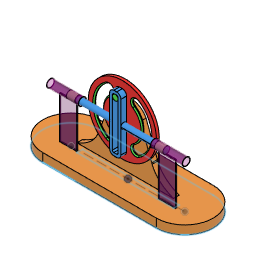
SCOTCH YOKE MECHANISM (Autodesk Fusion 360 design; units mm, degrees)
Autodesk Fusion 360 part; units mm, degrees
note: some values were not read from the file. Chosen so that the rebuilt part matches the saved one: that a step has no effect; which face or edge a step refers to; which pieces of a blend or face edit are solid. Set by a fixed rule: which sketch regions a step uses.
sketch "Holder stand" plane through (0, 0, 0) normal (0, 1, 0) x (1, 0, 0) in component "Holder stand"
  line L0 (-100, -50) -> (100, -50)
  arc A0 (100, -50) -> (100, 50) centre (100, 0) ccw
  line L1 (100, 50) -> (-100, 50)
  arc A1 (-100, 50) -> (-100, -50) centre (-100, 0) ccw
  line L2 (-100, 0) -> (100, 0) construction
  constraint tangent L0 A0
  constraint tangent A0 L1
  constraint parallel L0 L1
  constraint tangent L1 A1
  constraint tangent L0 A1
  constraint horizontal L2
  constraint midpoint L2 origin
extrude "Extrude1" add sketch "Holder stand" along normal blind 15 makes body 1 in component "Holder stand"
sketch "Crank holder hole" plane through (0, 0, 0) normal (0, 1, 0) x (1, 0, 0) in component "Holder stand"
  line L0 (-85, -5) -> (85, -5)
  line L1 (85, -5) -> (85, 5)
  line L2 (85, 5) -> (-85, 5)
  line L3 (-85, 5) -> (-85, -5)
  constraint horizontal L0
  constraint vertical L1
  constraint horizontal L2
  constraint vertical L3
extrude "Extrude2" cut sketch "Crank holder hole" along normal blind 15 bodies 1 in component "Holder stand"
sketch "Holder" plane through (0, 0, 0) normal (0, 0, 1) x (1, 0, 0) in component " Crank Holder"
  line L0 (0, 15) -> (0, 100.6882)
  line L1 (-26.793, 103.552) -> (-47.4731, 48.405)
  line L2 (-60, 15) -> (0, 15)
  line L3 (-60, 15) -> (-85, 15)
  spline S0 degree 5 poles (-85, 15) (-82.4129, 16.0125) (-77.423, 18.1587) (-70.4912, 21.7416) (-62.3731, 27.258) (-55.1239, 34.5502) (-50.7724, 41.0341) (-48.3509, 46.0734) (-47.1533, 49.2041) (-46.8071, 50.181) knots 0 0 0 0 0 0 0.1 0.2 0.3 0.4 0.444391 0.444391 0.444391 0.444391 0.444391 0.444391
  line L4 (-48.7805, 44.6118) -> (-44.8337, 55.7502)
  line L5 (26.793, 103.552) -> (47.4731, 48.405)
  spline S1 degree 5 poles (85, 15) (82.4129, 16.0125) (77.423, 18.1587) (70.4912, 21.7416) (62.3731, 27.258) (55.1239, 34.5502) (50.7724, 41.0341) (48.3509, 46.0734) (47.1533, 49.2041) (46.8071, 50.181) knots 0 0 0 0 0 0 0.1 0.2 0.3 0.4 0.444391 0.444391 0.444391 0.444391 0.444391 0.444391
  line L6 (-91.3253, 12.5245) -> (-78.6747, 17.4755)
  line L7 (91.3253, 12.5245) -> (78.6747, 17.4755)
  line L8 (48.7805, 44.6118) -> (44.8337, 55.7502)
  line L9 (60, 15) -> (0, 15)
  line L10 (60, 15) -> (85, 15)
  arc A0 (29.0974, 97.4069) -> (-29.0974, 97.4069) centre (0, 90) ccw
  point P0 (-46.8073, 50.1805)
  point P1 (46.8073, 50.1805)
  constraint vertical L0
  constraint perpendicular L0 L2
  constraint coincident L1 P0
  constraint parallel L2 L3
  constraint coincident L1 S0.end
  constraint midpoint S0.end L4
  constraint coincident S0 L1.end
  constraint midpoint L3.end L6
  constraint symmetric L2.end L0 L9.end
  constraint symmetric L0 L2.start L9.start
  constraint symmetric L0 L3.end S1.start
  constraint symmetric L0 P0 P1
  constraint symmetric L0 S0.end S1.end
  constraint symmetric L0 L4.start L8.start
  constraint symmetric L0 L4.end L8.end
  constraint symmetric L0 L1.end L5.end
  constraint symmetric L0 L6.start L7.start
  constraint symmetric L0 L6.end L7.end
  constraint coincident L0 A0.centre
  constraint coincident L1.start A0
  constraint coincident L5.start A0
  constraint coincident L5 A0.start
  constraint coincident L1 A0.end
extrude "Extrude1'" add sketch "Holder" along normal mid plane 10 separate body contours L1 L2 L3 S0 L5 S1 L9 L10 A0 makes body 2 in component " Crank Holder"
extrude "Extrude2'" add 1 faces at (-28.3333, 15, 1.6667) along direction (0, -1, 0) blind 15 on bodies 2 bodies 2 in component " Crank Holder"
sketch "Crank" plane through (0, 0, 5) normal (0, 0, 1) x (1, 0, 0) in component "Crank"
  spline S0 degree 5 poles (85, 15) (82.4129, 16.0125) (77.423, 18.1587) (70.4912, 21.7416) (62.3731, 27.258) (55.3901, 34.2824) (51.1876, 40.4215) (48.8448, 45.0699) (47.7125, 47.8006) (47.4731, 48.405) knots 0 0 0 0 0 0 0.1 0.2 0.3 0.4 0.428073 0.428073 0.428073 0.428073 0.428073 0.428073
  spline S1 degree 5 poles (47.4731, 48.405) (47.334, 48.7563) (47.1978, 49.1095) (47.0646, 49.4647) (46.9344, 49.8219) (46.8071, 50.181) knots 0.428073 0.428073 0.428073 0.428073 0.428073 0.428073 0.444391 0.444391 0.444391 0.444391 0.444391 0.444391
  line L0 (46.8071, 50.181) -> (26.793, 103.552)
  arc A0 (26.793, 103.552) -> (-26.793, 103.552) centre (0, 90) ccw
  line L1 (-26.793, 103.552) -> (-46.8071, 50.181)
  spline S2 degree 5 poles (-46.8071, 50.181) (-46.9344, 49.8219) (-47.0646, 49.4647) (-47.1978, 49.1095) (-47.334, 48.7563) (-47.4731, 48.405) knots -0.444391 -0.444391 -0.444391 -0.444391 -0.444391 -0.444391 -0.428073 -0.428073 -0.428073 -0.428073 -0.428073 -0.428073
  spline S3 degree 5 poles (-47.4731, 48.405) (-47.7125, 47.8006) (-48.8448, 45.0699) (-51.1876, 40.4215) (-55.3901, 34.2824) (-62.3731, 27.258) (-70.4912, 21.7416) (-77.423, 18.1587) (-82.4129, 16.0125) (-85, 15) knots -0.428073 -0.428073 -0.428073 -0.428073 -0.428073 -0.428073 -0.4 -0.3 -0.2 -0.1 0 0 0 0 0 0
  line L2 (-85, 15) -> (-85, 0)
  line L3 (-85, 0) -> (85, 0)
  line L4 (85, 0) -> (85, 15)
  circle A1 centre (0, 95) radius 60
  arc A2 (50, 95) -> (28.0513, 136.3899) centre (0, 95) ccw
  arc A3 (28.0513, 53.6101) -> (50, 95) centre (0, 95) ccw
  arc A4 (19.6359, 66.027) -> (35, 95) centre (0, 95) ccw
  arc A5 (35, 95) -> (19.6359, 123.973) centre (0, 95) ccw
  line L5 (16.99, 133.2275) -> (16.99, 133.2275)
  line L6 (16.99, 56.7725) -> (16.99, 56.7725)
  arc A6 (16.99, 133.2275) -> (19.6359, 123.973) centre (23.8436, 130.1814) ccw
  arc A7 (28.0513, 136.3899) -> (16.99, 133.2275) centre (23.8436, 130.1814) ccw
  arc A8 (19.6359, 66.027) -> (16.99, 56.7725) centre (23.8436, 59.8186) ccw
  arc A9 (16.99, 56.7725) -> (28.0513, 53.6101) centre (23.8436, 59.8186) ccw
  arc A10 (-16.99, 133.2275) -> (-28.0513, 136.3899) centre (-23.8436, 130.1814) ccw
  arc A11 (-19.6359, 123.973) -> (-16.99, 133.2275) centre (-23.8436, 130.1814) ccw
  arc A12 (-19.6359, 123.973) -> (-35, 95) centre (0, 95) ccw
  arc A13 (-28.0513, 136.3899) -> (-50, 95) centre (0, 95) ccw
  arc A14 (-50, 95) -> (-28.0513, 53.6101) centre (0, 95) ccw
  arc A15 (-35, 95) -> (-19.6359, 66.027) centre (0, 95) ccw
  arc A16 (-28.0513, 53.6101) -> (-16.99, 56.7725) centre (-23.8436, 59.8186) ccw
  arc A17 (-16.99, 56.7725) -> (-19.6359, 66.027) centre (-23.8436, 59.8186) ccw
  dimension "d26" = 7.5
  dimension "d27" = 7.5
  dimension "d28" = 7.5
  dimension "d29" = 7.5
  constraint concentric A3 A4
  constraint concentric A2 A5
  constraint tangent A4 A5
  constraint tangent A5 A6
  constraint tangent A2 A7
  constraint tangent A4 A8
  constraint tangent A3 A9
  measures "d26" radius of A6
  measures "d27" radius of A7
  measures "d28" radius of A8
  measures "d29" radius of A9
extrude "Extrude2''" add sketch "Crank" along normal blind 5 separate body contours L0 A0 L1 A1 A3 A4 A8 A9 A14 A15 A16 A17 | L0 A0 L1 A1 A2 A3 A4 A5 A6 A7 A10 A11 A12 A13 A14 A15 makes body 3 in component "Crank"
sketch "Crank Holder" plane through (0, 0, 5) normal (0, 0, 1) x (1, 0, 0) in component " Crank Holder"
  circle A0 centre (0, 95) radius 4.7
extrude "Extrude3" add sketch "Crank Holder" along normal blind 13 bodies 2 in component " Crank Holder"
sketch "Crank holder" plane through (0, 0, 10) normal (0, 0, 1) x (1, 0, 0) in component "Crank"
  arc A0 (19.6359, 66.027) -> (28.0513, 53.6101) centre (23.8436, 59.8186) ccw
  arc A1 (19.6359, 66.027) -> (19.6359, 123.973) centre (0, 95) ccw
  arc A2 (28.0513, 136.3899) -> (19.6359, 123.973) centre (23.8436, 130.1814) ccw
  arc A3 (28.0513, 53.6101) -> (28.0513, 136.3899) centre (0, 95) ccw
  arc A4 (-19.6359, 123.973) -> (-28.0513, 136.3899) centre (-23.8436, 130.1814) ccw
  arc A5 (-19.6359, 123.973) -> (-19.6359, 66.027) centre (0, 95) ccw
  arc A6 (-28.0513, 53.6101) -> (-19.6359, 66.027) centre (-23.8436, 59.8186) ccw
  arc A7 (-28.0513, 136.3899) -> (-28.0513, 53.6101) centre (0, 95) ccw
  circle A8 centre (0, 95) radius 60
  circle A9 centre (0, 95) radius 5
  constraint concentric A1 A9
extrude "Extrude3'" cut sketch "Crank holder" against normal blind 23 contours A9 bodies 3 in component "Crank"
sketch "Slider central part" plane through (0, 0, 10) normal (0, 0, 1) x (1, 0, 0) in component "Slider"
  line L0 (2.5, 145) -> (-2.5, 145)
  line L1 (-10, 137.5) -> (-10, 52.5)
  line L2 (-2.5, 45) -> (2.5, 45)
  line L3 (10, 52.5) -> (10, 137.5)
  arc A0 (-2.5, 145) -> (-10, 137.5) centre (-2.5, 137.5) ccw
  arc A1 (10, 137.5) -> (2.5, 145) centre (2.5, 137.5) ccw
  arc A2 (-10, 52.5) -> (-2.5, 45) centre (-2.5, 52.5) ccw
  arc A3 (2.5, 45) -> (10, 52.5) centre (2.5, 52.5) ccw
  arc A4 (-5, 52.5) -> (-2.5, 50) centre (-2.5, 52.5) ccw
  line L4 (-2.5, 50) -> (2.5, 50)
  arc A5 (2.5, 50) -> (5, 52.5) centre (2.5, 52.5) ccw
  line L5 (5, 52.5) -> (5, 137.5)
  arc A6 (5, 137.5) -> (2.5, 140) centre (2.5, 137.5) ccw
  line L6 (2.5, 140) -> (-2.5, 140)
  arc A7 (-2.5, 140) -> (-5, 137.5) centre (-2.5, 137.5) ccw
  line L7 (-5, 137.5) -> (-5, 52.5)
  point P0 (0, 95)
  dimension "d36" = 7.5
  dimension "d37" = 7.5
  dimension "d38" = 7.5
  dimension "d39" = 7.5
  dimension "d40" = -5
  constraint horizontal L0
  constraint perpendicular L0 L1
  constraint parallel L0 L2
  constraint parallel L1 L3
  constraint tangent L0 A0
  constraint tangent L1 A0
  constraint tangent L0 A1
  constraint tangent L3 A1
  constraint tangent L1 A2
  constraint tangent L2 A2
  constraint tangent L2 A3
  constraint tangent L3 A3
  measures "d36" radius of A0
  measures "d37" radius of A1
  measures "d38" radius of A2
  measures "d39" radius of A3
extrude "Extrude4" cut 1 faces at (1.1484, 93.4674, 18) along direction (0, 0, -1) up to surface (8 mm away) on bodies 2 bodies 2 in component " Crank Holder"
extrude "Extrude1''" add sketch "Slider central part" along normal blind 7.5 separate body makes body 4 in component "Slider"
extrude "Extrude2'''" cut 1 faces at (-8.3333, 109.1667, 10) along direction (0, 0, 1) blind 2.5 on bodies 4 bodies 4 in component "Slider"
extrude "Extrude7" add 1 faces at (-8.3333, 109.1667, 17.5) along direction (0, 0, 1) blind 5 on bodies 4 bodies 4 in component "Slider"
sketch "right smaller" plane through (10, 0, 0) normal (1, 0, 0) x (0, 0, -1) in component "Slider"
  line L0 (-12.5, 52.5) -> (-12.5, 137.5)
  line L1 (-12.5, 137.5) -> (-22.5, 137.5)
  line L2 (-22.5, 137.5) -> (-22.5, 52.5)
  line L3 (-22.5, 52.5) -> (-12.5, 52.5)
  line L4 (-17.5, 144.9359) -> (-17.5, 45)
  circle A0 centre (-17.5, 94.9679) radius 5.0001
  constraint perpendicular L1 L4
  constraint midpoint L4 A0.centre
extrude "Extrude8" add sketch "right smaller" along normal blind 60 contours L4 A0 | L4 A0 bodies 4 in component "Slider"
sketch "left smaller" plane through (-10, 0, 0) normal (-1, 0, 0) x (0, 0, 1) in component "Slider"
  line L0 (12.5, 137.5) -> (12.5, 52.5)
  line L1 (12.5, 52.5) -> (22.5, 52.5)
  line L2 (22.5, 52.5) -> (22.5, 137.5)
  line L3 (22.5, 137.5) -> (12.5, 137.5)
  circle A0 centre (17.499, 95.1) radius 5.001
  dimension "d78" = 10.002
  constraint tangent L2 A0
  measures "d78" diameter of A0
extrude "Extrude9" add sketch "left smaller" along normal blind 60 contours A0 bodies 4 in component "Slider"
sketch "right bigger" plane through (70, 0, 0) normal (1, 0, 0) x (0, 0, -1) in component "Slider"
  line L0 (-12.5, 94.9359) -> (-12.5, 95)
  arc A0 (-12.5, 95) -> (-22.5, 95) centre (-17.5, 94.9679) ccw
  line L1 (-22.5, 95) -> (-22.5, 94.9359)
  arc A1 (-22.5, 94.9359) -> (-12.5, 94.9359) centre (-17.5, 94.9679) ccw
  circle A2 centre (-17.5, 94.9679) radius 6.25
  dimension "d63" = 12.5
  constraint concentric A0 A2
  measures "d63" diameter of A2
extrude "Extrude10" add sketch "right bigger" along normal blind 15 contours L0 A0 L1 A1 | A2 bodies 4 in component "Slider"
sketch "left bigger" plane through (-70, 0, 0) normal (-1, 0, 0) x (0, 0, 1) in component "Slider"
  circle A0 centre (17.499, 95.1) radius 5.001
  circle A1 centre (17.499, 95.1) radius 6.25
  dimension "d66" = 12.5
  constraint concentric A0 A1
  measures "d66" diameter of A1
extrude "Extrude11" add sketch "left bigger" along normal blind 15 contours A0 | A1 bodies 4 in component "Slider"
sketch "Slider holder" plane through (0, 0, 10) normal (0, 0, 1) x (1, 0, 0) in component "Crank"
  circle A0 centre (0, 95) radius 5
  arc A1 (19.6359, 66.027) -> (28.0513, 53.6101) centre (23.8436, 59.8186) ccw
  arc A2 (19.6359, 66.027) -> (19.6359, 123.973) centre (0, 95) ccw
  arc A3 (28.0513, 136.3899) -> (19.6359, 123.973) centre (23.8436, 130.1814) ccw
  arc A4 (28.0513, 53.6101) -> (28.0513, 136.3899) centre (0, 95) ccw
  arc A5 (-19.6359, 123.973) -> (-28.0513, 136.3899) centre (-23.8436, 130.1814) ccw
  arc A6 (-19.6359, 123.973) -> (-19.6359, 66.027) centre (0, 95) ccw
  arc A7 (-28.0513, 53.6101) -> (-19.6359, 66.027) centre (-23.8436, 59.8186) ccw
  arc A8 (-28.0513, 136.3899) -> (-28.0513, 53.6101) centre (0, 95) ccw
  circle A9 centre (0, 95) radius 60
  circle A10 centre (0, 95) radius 35
  circle A11 centre (0, 95) radius 50
  circle A12 centre (0, 135) radius 4.97
  constraint concentric A0 A10
  constraint concentric A10 A11
extrude "Extrude4'" add sketch "Slider holder" along normal up to surface (12.5 mm away) contours A12 bodies 3 in component "Crank"
sketch "Left part" plane through (-10, 0, 0) normal (-1, 0, 0) x (0, 0, 1) in component "Slider holder"
  arc A0 (12.5, 94.9586) -> (22.5, 95.1) centre (17.499, 95.1) ccw
  line L0 (12.5, 94.9586) -> (12.5, 52.5)
  line L1 (12.5, 52.5) -> (22.5, 52.5)
  line L2 (22.5, 52.5) -> (22.5, 95.1)
  circle A1 centre (17.499, 95.1) radius 6.25
  circle A2 centre (17.499, 95.1) radius 7
  dimension "d71" = 12.5
  dimension "d72" = 14
  constraint concentric A0 A1
  constraint concentric A1 A2
  measures "d71" diameter of A1
  measures "d72" diameter of A2
extrude "Extrude1'''" add sketch "Left part" along normal blind 90 separate body contours L0 L2 A1 A2 | L0 L2 A1 A2 makes body 5 in component "Slider holder"
extrude "Extrude2''''" cut 1 faces at (-10, 90.8409, 12.2814) along direction (-1, 0, 0) blind 54 on bodies 5 bodies 5 in component "Slider holder"
move_face "OffsetFaces1" offset -0.2 1 faces at (-80, 94.4777, 23.7179) on bodies 4 in component "Slider"
sketch "Right part" plane through (10, 0, 0) normal (1, 0, 0) x (0, 0, -1) in component "Slider holder"
  arc A0 (-12.5, 95) -> (-22.5, 95) centre (-17.5, 94.9679) ccw
  line L0 (-12.5, 95) -> (-12.5, 137.5)
  line L1 (-12.5, 137.5) -> (-22.5, 137.5)
  line L2 (-22.5, 137.5) -> (-22.5, 95)
  circle A1 centre (-17.5, 94.9679) radius 6.25
  circle A2 centre (-17.5, 94.9679) radius 7
  dimension "d79" = 12.5
  dimension "d80" = 14
  constraint concentric A0 A1
  constraint concentric A0 A2
  measures "d79" diameter of A1
  measures "d80" diameter of A2
extrude "Extrude3''" add sketch "Right part" along normal blind 80 separate body contours L0 L2 A1 A2 | L0 L2 A1 A2 makes body 6 in component "Slider holder"
extrude "Extrude4''" add 1 faces at (90, 99.2258, 22.7186) along direction (1, 0, 0) blind 10 on bodies 6 bodies 6 in component "Slider holder"
extrude "Extrude5" cut 1 faces at (10, 94.6202, 10.7761) along direction (1, 0, 0) blind 54 on bodies 6 bodies 6 in component "Slider holder"
move_face "OffsetFaces2" offset -0.2 1 faces at (80, 95.2795, 11.2578) on bodies 4 in component "Slider"
sketch "Connector to holder stand" plane through (0, 15, 0) normal (0, 1, 0) x (-1, 0, 0) in component "Slider holder"
  line L0 (85, -5) -> (-85, -5)
  line L1 (-85, -5) -> (-85, 5)
  line L2 (-85, 5) -> (85, 5)
  line L3 (85, 5) -> (85, -5)
  arc A0 (100, -50) -> (100, 50) centre (100, 0) ccw
  line L4 (100, 50) -> (-100, 50)
  arc A1 (-100, 50) -> (-100, -50) centre (-100, 0) ccw
  line L5 (-100, -50) -> (100, -50)
  line L6 (72.0384, 18.4939) -> (92.0384, 18.4939)
  line L7 (92.0384, 18.4939) -> (92.0384, 16.4939)
  line L8 (92.0384, 16.4939) -> (72.0384, 16.4939)
  line L9 (72.0384, 16.4939) -> (72.0384, 18.4939)
  line L10 (72.0384, 18.4939) -> (92.0384, 16.4939) construction
  line L11 (92.0384, 18.4939) -> (72.0384, 16.4939) construction
  line L12 (0, -140) -> (0, 145)
  line L13 (-92.0384, 18.4939) -> (-72.0384, 16.4939) construction
  line L14 (-72.0384, 18.4939) -> (-92.0384, 18.4939)
  line L15 (-72.0384, 18.4939) -> (-92.0384, 16.4939) construction
  line L16 (-92.0384, 16.4939) -> (-72.0384, 16.4939)
  line L17 (-92.0384, 18.4939) -> (-92.0384, 16.4939)
  line L18 (-72.0384, 16.4939) -> (-72.0384, 18.4939)
  point P0 (82.0384, 17.4939)
  point P1 (-82.0384, 17.4939)
  dimension "d88" = 20
  dimension "d89" = 2
  constraint horizontal L6
  constraint perpendicular L6 L7
  constraint parallel L6 L8
  constraint parallel L7 L9
  constraint coincident L10 P0
  constraint coincident L11 P0
  constraint vertical L12
  constraint symmetric L6.start L12 L14.start
  constraint symmetric L6.end L12 L13.start
  constraint symmetric L7.end L12 L15.end
  constraint symmetric L8.end L12 L13.end
  constraint symmetric P0 L12 P1
  measures "d88" distance of L7.end L8.end
  measures "d89" distance of L6.end L7.end
extrude "Extrude3'''" cut sketch "Connector to holder stand" against normal blind 20 contours L6 L7 L8 L9 | L14 L16 L17 L18 bodies 1 in component "Holder stand"
extrude "Extrude6" add sketch "Connector to holder stand" along normal up to surface separate body contours L6 L7 L8 L9 end surface at (-76, 95.797, 24.4642) on bodies 5 makes body 7 in component "Slider holder"
extrude "Extrude7'" add sketch "Connector to holder stand" along normal up to surface separate body contours L14 L16 L17 L18 end surface at (88, 95.6649, 10.5348) on bodies 6 makes body 8 in component "Slider holder"
extrude "Extrude8'" add 2 faces at (-78.7051, 15, 17.8273) (85.3718, 15, 17.8273) along direction (0, -1, 0) blind 15 on bodies 7 8 bodies 7 8 in component "Slider holder"
sketch "Left closing" plane through (-100, 0, 0) normal (-1, 0, 0) x (0, 0, 1) in component "Slider holder"
  circle A0 centre (17.499, 95.1) radius 6.25
  circle A1 centre (17.499, 95.1) radius 7
  circle A2 centre (17.499, 95.1) radius 7
  constraint concentric A0 A2
extrude "Extrude9'" add sketch "Left closing" against normal blind 0.5 contours A0 | A1 A2 bodies 5 in component "Slider holder"
sketch "Right closing" plane through (100, 0, 0) normal (1, 0, 0) x (0, 0, -1) in component "Slider holder"
  circle A0 centre (-17.5, 94.9679) radius 6.25
  circle A1 centre (-17.5, 94.9679) radius 7
  circle A2 centre (-17.5, 94.9679) radius 7
  constraint concentric A0 A2
extrude "Extrude10'" add sketch "Right closing" against normal blind 0.5 contours A0 | A1 A2 bodies 6 in component "Slider holder"
fillet "Fillet1" radius 2 16 edges at (-50, 95, 10) (-17.6351, 134.3891, 10) (-35, 95, 10) (-17.6351, 55.6109, 10) (17.6351, 134.3891, 10) (50, 95, 10) (17.6351, 55.6109, 10) (35, 95, 10) (-17.6351, 55.6109, 5) (-50, 95, 5) (-17.6351, 134.3891, 5) (-35, 95, 5) (17.6351, 134.3891, 5) (50, 95, 5) (17.6351, 55.6109, 5) (35, 95, 5) on bodies 3 in component "Crank"
extrude "Extrude11'" cut 1 faces at (-100, 97.3748, 16.9798) along direction (1, 0, 0) blind 2 on bodies 5 bodies 5 in component "Slider holder"
extrude "Extrude12" add 1 faces at (-98, 94.4417, 24.1997) along direction (-1, 0, 0) blind 22 on bodies 5 bodies 5 in component "Slider holder"
extrude "Extrude13" cut 1 faces at (100, 97.14, 16.6475) along direction (-1, 0, 0) blind 2 on bodies 6 bodies 6 in component "Slider holder"
extrude "Extrude14" add 1 faces at (98, 90.1396, 22.1925) along direction (1, 0, 0) blind 22 on bodies 6 bodies 6 in component "Slider holder"
extrude "Extrude15" add 1 faces at (-92.0384, 29.3693, 17.6054) along direction (-1, 0, 0) blind 5 on bodies 7 bodies 7 5 in component "Slider holder"
extrude "Extrude16" add 1 faces at (92.0384, 29.3252, 17.6053) along direction (1, 0, 0) blind 10 on bodies 8 bodies 8 6 in component "Slider holder"
extrude "Extrude17" add 1 faces at (-97.0384, 29.3693, 17.6054) along direction (-1, 0, 0) blind 5 on bodies 7 bodies 7 in component "Slider holder"
extrude "Extrude4'''" cut 1 faces at (-92.0384, 10, 17.8273) along direction (-1, 0, 0) blind 10 on bodies 1 bodies 1 in component "Holder stand"
extrude "Extrude5'" cut 1 faces at (92.0384, 10, 17.8273) along direction (1, 0, 0) blind 10 on bodies 1 bodies 1 in component "Holder stand"
move_face "MoveFace1" [no effect] in component "Slider holder"
copy_body "CopyPasteBodies1" bodies 7 makes body 9 in component "Slider holder"
move_body "Move1" bodies 9 to x (1, 0, 0) y (0, 1, 0) z (0, 0, 1) at (-65, 0, 0) in component "Slider holder"
delete_face "DeleteFace1" 1 faces at (-95.3461, 88.4062, 19.5467) on bodies 7 in component "Slider holder"
delete_face "DeleteFace2" 1 faces at (-147.0384, 58.7807, 18.4939) on bodies 9 in component "Slider holder"
move_body "Move2" bodies 9 to x (1, 0, 0) y (0, 1, 0) z (0, 0, 1) at (66, 0, 0) in component "Slider holder"
copy_body "CopyPasteBodies2" bodies 8 makes body 10 in component "Slider holder"
move_body "Move3" bodies 10 to x (1, 0, 0) y (0, 1, 0) z (0, 0, 1) at (70, 0, 0) in component "Slider holder"
delete_face "DeleteFace3" 1 faces at (95.3461, 88.274, 19.5474) on bodies 8 in component "Slider holder"
delete_face "DeleteFace4" 1 faces at (152.0384, 29.3463, 18.4939) on bodies 10 in component "Slider holder"
move_body "Move4" bodies 10 to x (1, 0, 0) y (0, 1, 0) z (0, 0, 1) at (-70, 0, 0) in component "Slider holder"
component "Holder stand" placed x (1, 0, 0) y (0, 1, 0) z (0, 0, 1) at (0, 0, 0)
component "Crank" placed x (1, 0, 0) y (0, 1, 0) z (0, 0, 1) at (0, 0, 0)
component " Crank Holder" placed x (1, 0, 0) y (0, 1, 0) z (0, 0, 1) at (0, 0, 0)
component "Slider" placed x (1, 0, 0) y (0, 1, 0) z (0, 0, 1) at (0, 0, 0)
component "Slider holder" placed x (1, 0, 0) y (0, 1, 0) z (0, 0, 1) at (0, 0, 0)
named bodies: "Holder Stand", "Crank holder", "Crank", "Slider", "Left part", "right part", "Left holder stand", "Right holder stand", "Left holder", "Right holder"
